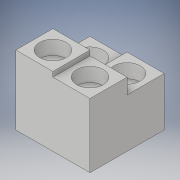
# Autodesk Inventor part: screwprint
Saved by Autodesk Inventor 2019 (Build 230136000, 136)
## iProperties
Created: 2018-12-19
Part Number: screwprint
Material: Generic
Document SubType Name: Modeling
Designer: assman
Density: 1 g/cm^3
Appearance: Default
Author: assman
## iProperties of the stored document screwprint_3DPrint.ipt
Created: 2018-12-19
Part Number: screwprint_3DPrint
Material: Generic
Document SubType Name: Modeling
Designer: assman
Density: 1 g/cm^3
Appearance: Default
Author: assman
Autodesk Inventor part; units mm, degrees
ref_plane "YZ Plane" through (0, 0, 0) normal (1, 0, 0) x (0, 1, 0)
ref_plane "XZ Plane" through (0, 0, 0) normal (0, 1, 0) x (-1, 0, 0)
ref_plane "XY Plane" through (0, 0, 0) normal (0, 0, 1) x (1, 0, 0)
sketch "Sketch1" plane through (0, 0, 0) normal (0, 1, 0) x (-1, 0, 0)
  line L0 (15, 15) -> (0, 15)
  line L1 (0, 15) -> (0, 0)
  line L2 (0, 0) -> (15, 0)
  line L3 (15, 0) -> (15, 15)
  dimension "d0" = 15
  dimension "d1" = 15
  constraints: 8 end point, 2 parallel, 1 coincident, 1 horizontal, 1 perpendicular
  measures "d0" distance of L2.end L1.end
  measures "d1" distance of L1.end L0.end
extrude "Extrusion1" add sketch "Sketch1" along normal blind 13
sketch "Sketch2" plane through (0, 13, 0) normal (0, 1, 0) x (1, 0, 0)
  line L0 (-15, -15) -> (0, -15) construction
  line L1 (0, -15) -> (0, 0) construction
  line L2 (0, 0) -> (-15, 0) construction
  line L3 (-15, 0) -> (-15, -15) construction
  line L4 (-15, 0) -> (-15, -15) construction
  line L5 (-15, -7.5) -> (0, -7.5) construction
  line L6 (-15, -7.5) -> (0, -7.5)
  line L7 (0, -7.5) -> (0, 0)
  line L8 (0, 0) -> (-15, 0)
  line L9 (-15, 0) -> (-15, -7.5)
  constraints: 10 end point, 2 midpoint, 2 parallel, 1 horizontal, 1 perpendicular
extrude "Extrusion2" cut sketch "Sketch2" against normal blind 4.1
sketch "Sketch3" plane through (0, 13, 0) normal (0, 1, 0) x (1, 0, 0)
  line L0 (0, -7.5) -> (-15, -7.5) construction
  line L1 (-15, -7.5) -> (-15, -15) construction
  line L2 (-15, -15) -> (0, -15) construction
  line L3 (0, -15) -> (0, -7.5) construction
  line L4 (-15, -15) -> (0, -15) construction
  line L5 (-7.5, -15) -> (-7.5, -7.5) construction
  line L6 (-15, -15) -> (-7.5, -15)
  line L7 (-7.5, -15) -> (-7.5, -7.5)
  line L8 (-7.5, -7.5) -> (-15, -7.5)
  line L9 (-15, -7.5) -> (-15, -15)
  point P0 (0, 0)
  constraints: 10 end point, 2 midpoint, 2 parallel, 1 horizontal, 1 perpendicular
extrude "Extrusion3" add sketch "Sketch3" along normal blind 1
sketch "Sketch4" plane through (0, 8.9, 0) normal (0, 1, 0) x (1, 0, 0)
  line L0 (0, 0) -> (0, -7.5) construction
  line L1 (-15, 0) -> (0, 0) construction
  line L2 (-15, -7.5) -> (-15, 0) construction
  line L3 (0, -7.5) -> (-15, -7.5) construction
  line L4 (-7.5, -7.5) -> (-7.5, 0) construction
  line L5 (-7.5, -7.5) -> (0, -7.5)
  line L6 (0, -7.5) -> (0, 0)
  line L7 (0, 0) -> (-7.5, 0)
  line L8 (-7.5, 0) -> (-7.5, -7.5)
  constraints: 10 end point, 2 midpoint, 2 parallel, 1 horizontal, 1 perpendicular
extrude "Extrusion4" add sketch "Sketch4" along normal blind 1
sketch "Sketch5" plane through (0, 14, 0) normal (0, 1, 0) x (1, 0, 0)
  line L0 (-15, -15) -> (-7.5, -15) construction
  line L1 (-7.5, -15) -> (-7.5, -7.5) construction
  line L2 (-7.5, -7.5) -> (-15, -7.5) construction
  line L3 (-15, -7.5) -> (-15, -15) construction
  point P0 (0, 0)
  point P1 (-11.25, -11.25)
  point P2 (-11.25, -11.25)
  constraints: 1 coincident
sketch "Sketch6" plane through (0, 13, 0) normal (0, 1, 0) x (1, 0, 0)
  line L0 (-7.5, -7.5) -> (-7.5, -15) construction
  line L1 (-7.5, -15) -> (0, -15) construction
  line L2 (0, -15) -> (0, -7.5) construction
  line L3 (0, -7.5) -> (-7.5, -7.5) construction
  point P0 (0, 0)
  point P1 (-3.75, -11.25)
sketch "Sketch7" plane through (0, 9.9, 0) normal (0, 1, 0) x (1, 0, 0)
  line L0 (0, -7.5) -> (0, 0) construction
  line L1 (0, 0) -> (-7.5, 0) construction
  line L2 (-7.5, 0) -> (-7.5, -7.5) construction
  line L3 (0, -7.5) -> (-7.5, -7.5) construction
  point P0 (-3.75, -3.75)
sketch "Sketch8" plane through (0, 8.9, 0) normal (0, 1, 0) x (1, 0, 0)
  line L0 (-7.5, -7.5) -> (-7.5, 0) construction
  line L1 (-15, 0) -> (-7.5, 0) construction
  line L2 (-15, -7.5) -> (-15, 0) construction
  line L3 (-7.5, -7.5) -> (-15, -7.5) construction
  point P0 (0, 0)
  point P1 (-11.25, -3.75)
hole "Hole1" at (-11.25, 14, 11.25) direction (0, -1, 0) diameter 2.4638 depth 13 counterbore diameter 5.37 counterbore depth 2.85
hole "Hole2" at (-3.75, 13, 11.25) direction (0, -1, 0) diameter 2.4638 depth 13 counterbore diameter 5.37 counterbore depth 2.85
hole "Hole3" at (-11.25, 8.9, 3.75) direction (0, -1, 0) diameter 2.4638 depth 8.9 counterbore diameter 5.37 counterbore depth 2.85
hole "Hole4" at (-3.75, 9.9, 3.75) direction (0, -1, 0) diameter 2.4638 depth 8.9 counterbore diameter 5.37 counterbore depth 2.85
body "Solid1"
